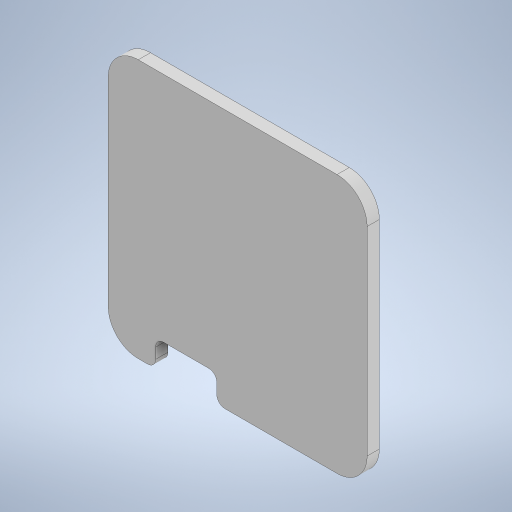
# Autodesk Inventor part: back cover
Saved by Autodesk Inventor 2023 (Build 270158000, 158)
## iProperties
Created: 2025-01-03
Part Number: back cover
Material: Generic
Document SubType Name: Modeling
Designer: jonwo
Density: 1 g/cm^3
Appearance: Default
Author: jonwo
Autodesk Inventor part; units mm, degrees
ref_plane "YZ Plane" through (0, 0, 0) normal (1, 0, 0) x (0, 1, 0)
ref_plane "Work Plane1" through (0, 0, 0) normal (0, 0, 1) x (1, 0, 0)
sketch "Sketch1" plane through (0, 0, 0) normal (0, 0, 1) x (1, 0, 0)
  line L0 (-8.0903, -30.4) -> (-17.1403, -30.4) projected
  line L1 (-17.1403, -30.4) -> (-17.1403, -26.8) projected
  line L2 (-17.1403, -26.8) -> (-8.0903, -26.8) projected
  line L3 (-8.0903, -26.8) -> (-8.0903, -30.4) projected
  line L4 (-24.384, -24.384) -> (-24.384, 18.034) projected
  arc A0 (-18.034, 24.384) -> (-24.384, 18.034) centre (-18.034, 18.034) ccw projected
  line L5 (-18.034, 24.384) -> (18.034, 24.384) projected
  arc A1 (24.384, 18.034) -> (18.034, 24.384) centre (18.034, 18.034) ccw projected
  line L6 (24.384, 18.034) -> (24.384, -18.034) projected
  arc A2 (18.034, -24.384) -> (24.384, -18.034) centre (18.034, -18.034) ccw projected
  line L7 (18.034, -24.384) -> (-24.384, -24.384) projected
  arc A3 (-31.75, -24.384) -> (-24.384, -31.75) centre (-24.384, -24.384) ccw projected
  line L8 (24.384, -31.75) -> (-24.384, -31.75) projected
  arc A4 (24.384, -31.75) -> (31.75, -24.384) centre (24.384, -24.384) ccw projected
  arc A5 (31.75, 24.384) -> (24.384, 31.75) centre (24.384, 24.384) ccw projected
  line L9 (-24.384, 31.75) -> (24.384, 31.75) projected
  arc A6 (-24.384, 31.75) -> (-31.75, 24.384) centre (-24.384, 24.384) ccw projected
  arc A7 (-31.75, 6) -> (-30.75, 5) centre (-30.75, 6) ccw projected
  line L10 (-30.75, 5) -> (-29.75, 5) projected
  arc A8 (-28.75, 4) -> (-29.75, 5) centre (-29.75, 4) ccw projected
  line L11 (-28.75, 4) -> (-28.75, -4) projected
  arc A9 (-29.75, -5) -> (-28.75, -4) centre (-29.75, -4) ccw projected
  line L12 (-29.75, -5) -> (-30.75, -5) projected
  arc A10 (-30.75, -5) -> (-31.75, -6) centre (-30.75, -6) ccw projected
  line L13 (-31.75, -24.384) -> (-31.75, -6) projected
  line L14 (31.75, -6) -> (31.75, -24.384) projected
  arc A11 (31.75, -6) -> (30.75, -5) centre (30.75, -6) ccw projected
  line L15 (30.75, -5) -> (29.75, -5) projected
  arc A12 (28.75, -4) -> (29.75, -5) centre (29.75, -4) ccw projected
  line L16 (28.75, -4) -> (28.75, 4) projected
  arc A13 (29.75, 5) -> (28.75, 4) centre (29.75, 4) ccw projected
  line L17 (29.75, 5) -> (30.75, 5) projected
  arc A14 (30.75, 5) -> (31.75, 6) centre (30.75, 6) ccw projected
  line L18 (31.75, 24.384) -> (31.75, 6) projected
  line L19 (-31.75, 6) -> (-31.75, 24.384) projected
  line L20 (-31.75, 6) -> (-31.75, -6)
  line L21 (31.75, 6) -> (31.75, -6)
  point P0 (0, 0)
  constraints: 4 end point, 1 vertical
extrude "Extrusion1" add sketch "Sketch1" along normal blind 3 contours L0 L1 L2 L3 | L4 A0 L5 A1 L6 A2 L7 | L13 A10 L12 A9 L11 A8 L10 A7 L19 A6 L9 A5 L18 A14 L17 A13 L16 A12 L15 A11 L14 A4 L8 A3 | L20 A7 L10 A8 L11 A9 L12 A10 | A11 L15 A12 L16 A13 L17 A14 L21
sketch "Sketch2" plane through (0, 0, 0) normal (0, 0, 1) x (1, 0, 0)
  line L0 (-24.384, -24.384) -> (-24.384, 18.034) projected
  arc A0 (-18.034, 24.384) -> (-24.384, 18.034) centre (-18.034, 18.034) ccw projected
  line L1 (-18.034, 24.384) -> (18.034, 24.384) projected
  arc A1 (24.384, 18.034) -> (18.034, 24.384) centre (18.034, 18.034) ccw projected
  line L2 (24.384, 18.034) -> (24.384, -18.034) projected
  arc A2 (18.034, -24.384) -> (24.384, -18.034) centre (18.034, -18.034) ccw projected
  line L3 (18.034, -24.384) -> (-24.384, -24.384) projected
  line L4 (-18.4403, -24.184) -> (-6.7903, -24.184) projected
  line L5 (-6.7903, -24.184) -> (-6.7903, -23.584) projected
  line L6 (-6.7903, -23.584) -> (-18.4403, -23.584) projected
  line L7 (-18.4403, -23.584) -> (-18.4403, -24.184) projected
  line L8 (-3.4903, -30.4) -> (-3.4903, -25.284) projected
  line L9 (-21.7403, -25.284) -> (-21.7403, -30.4) projected
  line L10 (-18.6403, -23.384) -> (-6.5903, -23.384)
  line L11 (-6.5903, -23.384) -> (-6.5903, -24.384)
  line L12 (-6.5903, -24.384) -> (-18.6403, -24.384)
  line L13 (-18.6403, -24.384) -> (-18.6403, -23.384)
  point P0 (-6.7903, -24.384)
  point P1 (-18.4403, -24.384)
  dimension "d4" = 0.2
  constraints: 8 end point, 2 point on line, 3 other
  measures "d4" distance between parallel lines of L6 L10
ref_plane "Work Plane2" through (-21.7403, -25.284, -2) normal (0, 0, -1) x (0, 1, 0)
extrude "Extrusion2" add sketch "Sketch2" against normal up to surface (2 mm away) contours L0 A0 L1 A1 L2 A2 L3 L11 L10 L13
sketch "Sketch3" plane through (18.034, 24.384, -2) normal (0, 0, -1) x (-1, 0, 0)
  line L0 (36.6743, -48.768) -> (36.6743, -47.768) projected
  line L1 (42.418, -48.768) -> (36.6743, -48.768) projected
  line L2 (42.418, -6.35) -> (42.418, -48.768) projected
  arc A0 (42.418, -6.35) -> (36.068, 0) centre (36.068, -6.35) ccw projected
  line L3 (0, 0) -> (36.068, 0) projected
  arc A1 (0, 0) -> (-6.35, -6.35) centre (0, -6.35) ccw projected
  line L4 (-6.35, -42.418) -> (-6.35, -6.35) projected
  arc A2 (-6.35, -42.418) -> (0, -48.768) centre (0, -42.418) ccw projected
  line L5 (24.6243, -48.768) -> (0, -48.768) projected
  line L6 (24.6243, -47.768) -> (24.6243, -48.768) projected
  line L7 (36.6743, -47.768) -> (24.6243, -47.768) projected
  line L8 (42.418, -6.35) -> (42.418, -48.768) projected
  line L9 (24.6243, -48.768) -> (0, -48.768) projected
  line L10 (18.034, -48.768) -> (0, -48.768)
  line L11 (42.418, -24.384) -> (42.418, -6.35)
  arc A3 (40.418, -6.35) -> (36.068, -2) centre (36.068, -6.35) ccw
  line L12 (36.068, -2) -> (0, -2)
  arc A4 (0, -2) -> (-4.35, -6.35) centre (0, -6.35) ccw
  line L13 (-4.35, -6.35) -> (-4.35, -42.418)
  arc A5 (-4.35, -42.418) -> (0, -46.768) centre (0, -42.418) ccw
  line L14 (40.418, -6.35) -> (40.418, -24.384)
  line L15 (0, -46.768) -> (18.034, -46.768)
  line L16 (18.034, -48.768) -> (18.034, -46.768)
  line L17 (42.418, -24.384) -> (40.418, -24.384)
  point P0 (18.034, -24.384)
  point P1 (18.034, -48.768)
  dimension "d9" = 2
  constraints: 16 end point, 6 point on circle, 3 centre point, 3 perpendicular, 3 point on line, 1 horizontal, 1 vertical, 4 other
  measures "d9" distance between parallel lines of L3 L12
extrude "Extrusion4" add sketch "Sketch3" along normal blind 4 contours L17 L14 A3 L12 A4 L13 A5 L15 L16 L5 A2 L4 A1 L3 A0 L2
chamfer "Chamfer1" distance 3 angle 45 7 edges at (0, 22.384, -2) (21.1099, 21.1099, -2) (22.384, 0, -2) (21.1099, -21.1099, -2) (9.017, -22.384, -2) (-21.1099, 21.1099, -2) (-22.384, 9.017, -2)
chamfer "Chamfer2" distance 0.6 angle 45 7 edges at (22.5241, -22.5241, -6) (9.017, -24.384, -6) (24.384, 0, -6) (22.5241, 22.5241, -6) (0, 24.384, -6) (-22.5241, 22.5241, -6) (-24.384, 9.017, -6)
sketch "Sketch4" plane through (0, 0, 3) normal (0, 0, 1) x (1, 0, 0)
  arc A0 (-15.8303, -27) -> (-17.0803, -28.25) centre (-15.8303, -28.25) ccw construction
  arc A1 (-16.7803, -28.96) -> (-15.8303, -29.91) centre (-15.8303, -28.96) ccw construction
  arc A2 (-9.3903, -30.21) -> (-8.1403, -28.96) centre (-9.3903, -28.96) ccw construction
  arc A3 (-8.1403, -28.25) -> (-9.3903, -27) centre (-9.3903, -28.25) ccw construction
  arc A4 (-17.0803, -28.96) -> (-15.8303, -30.21) centre (-15.8303, -28.96) ccw construction
  line L0 (-17.0803, -28.25) -> (-17.0803, -28.96) construction
  line L1 (-8.1403, -28.25) -> (-8.1403, -28.96) construction
  line L2 (-20.1103, -35.035) -> (-20.1103, -25.15)
  line L3 (-20.1103, -25.15) -> (-5.1103, -25.15)
  line L4 (-5.1103, -25.15) -> (-5.1103, -35.8505)
  line L5 (-24.384, -31.75) -> (24.384, -31.75) projected
  line L6 (-12.6103, -26.4828) -> (-12.6103, -30.7525) construction
  point P0 (0, 0)
  point P1 (-20.1103, -31.75)
  point P2 (-5.1103, -31.75)
  dimension "d18" = 6.6
  dimension "d20" = 15
  constraints: 12 end point, 3 vertical, 2 perpendicular, 1 parallel, 2 other
  measures "d18" distance between parallel lines of L5 L3
  measures "d20" distance between parallel lines of L4 L2
extrude "Extrusion5" cut sketch "Sketch4" against normal through all
fillet "Fillet1" radius 2 4 edges at (-20.1103, -25.15, 1.5) (-5.1103, -25.15, 1.5) (-20.1103, -31.75, 1.5) (-5.1103, -31.75, 1.5)
sketch "Sketch5" plane through (-6.5903, -23.384, -2) normal (0, 0, -1) x (-1, 0, 0)
  line L0 (16.1937, 2) -> (-6.2063, 2)
  line L1 (-6.2063, 2) -> (-6.2063, 10)
  line L2 (-6.2063, 10) -> (16.1937, 10)
  line L3 (16.1937, 10) -> (16.1937, 2)
  line L4 (0, -1) -> (-6.5903, -1) projected
  line L5 (17.7937, 23.384) -> (17.7937, -1) projected
  point P0 (-6.5903, 23.384)
  dimension "d4" = 0.2
  dimension "d24" = 3
  dimension "d25" = 24
  dimension "d26" = 1.6
  dimension "d27" = 8
  constraints: 8 end point, 2 parallel, 1 horizontal, 1 perpendicular
  measures "d24" distance between parallel lines of L4 L0
  measures "d25" distance between parallel lines of L1 L5
  measures "d26" distance between parallel lines of L5 L3
  measures "d27" distance between parallel lines of L0 L2
extrude "pcb clearance" cut sketch "Sketch5" against normal up to surface (2 mm away)
body "Solid1"
